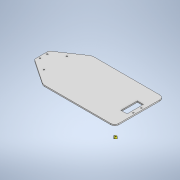
# Autodesk Inventor part: base
Saved by Autodesk Inventor 2020 (Build 240168000, 168)
## iProperties
Created: 2019-08-02
Part Number: base
Material: Generic
Document SubType Name: Modeling
Designer: n10208577
Density: 1 g/cm^3
Appearance: Default
Author: n10208577
Autodesk Inventor part; units mm, degrees
ref_plane "YZ Plane" through (0, 0, 0) normal (1, 0, 0) x (0, 1, 0)
ref_plane "XZ Plane" through (0, 0, 0) normal (0, 1, 0) x (-1, 0, 0)
ref_plane "XY Plane" through (0, 0, 0) normal (0, 0, 1) x (1, 0, 0)
sketch "Sketch1" plane through (0, 0, 0) normal (0, 1, 0) x (-1, 0, 0)
  line L0 (0, 0) -> (0, -28)
  line L1 (0, 0) -> (0, 28)
  circle A0 centre (0, 28) radius 1.6
  circle A1 centre (0, -28) radius 1.6
  line L2 (0, 0) -> (28.5, 0)
  line L3 (28.5, 0) -> (28.5, 8.75)
  line L4 (28.5, 0) -> (28.5, -8.75)
  circle A2 centre (28.5, 8.75) radius 1.6
  circle A3 centre (28.5, -8.75) radius 1.6
  line L5 (-200, 0) -> (-200, -10)
  line L6 (-200, 0) -> (-200, 10)
  circle A4 centre (-200, -10) radius 1.6
  circle A5 centre (-200, 10) radius 1.6
  line L7 (-200, 0) -> (-195, 0)
  line L8 (-195, 0) -> (-195, 20)
  line L9 (-195, 20) -> (-180, 20)
  line L10 (-180, 20) -> (-180, -20)
  line L11 (-180, -20) -> (-195, -20)
  line L12 (-195, -20) -> (-195, 0)
  line L13 (0, 0) -> (-180, 0)
  line L14 (-195, 0) -> (-200, 0)
  line L15 (-200, 0) -> (-205, 0)
  line L16 (-205, 0) -> (-205, 50)
  line L17 (28.5, 8.75) -> (0, 28)
  line L18 (-195, 60) -> (-34.1018, 60)
  line L19 (31.2986, 18.9271) -> (-25.706, 57.4302)
  line L20 (28.5, 8.75) -> (33.5, 8.75)
  line L21 (33.5, 14.7837) -> (33.5, -14.7837)
  line L22 (33.5, -8.75) -> (28.5, -8.75)
  line L23 (-205, 0) -> (-205, -50)
  line L24 (-195, -60) -> (-34.1018, -60)
  line L25 (31.2986, -18.9271) -> (-25.706, -57.4302)
  arc A6 (-25.706, 57.4302) -> (-34.1018, 60) centre (-34.1018, 45) ccw
  arc A7 (-34.1018, -60) -> (-25.706, -57.4302) centre (-34.1018, -45) ccw
  arc A8 (33.5, 14.7837) -> (31.2986, 18.9271) centre (28.5, 14.7837) ccw
  arc A9 (31.2986, -18.9271) -> (33.5, -14.7837) centre (28.5, -14.7837) ccw
  arc A10 (-205, -50) -> (-195, -60) centre (-195, -50) ccw
  arc A11 (-195, 60) -> (-205, 50) centre (-195, 50) ccw
  point P0 (-205, 60)
  point P1 (-29.5106, 60)
  point P2 (36.2986, 15.5499)
  point P3 (-205, -60)
  point P4 (-29.5106, -60)
  point P5 (36.2986, -15.5499)
  point P6 (-206.7664, -60)
  dimension "d0" = 28
  dimension "d1" = 28
  dimension "d2" = 3.2
  dimension "d3" = 3.2
  dimension "d4" = 28.5
  dimension "d5" = 8.75
  dimension "d6" = 8.75
  dimension "d7" = 3.2
  dimension "d8" = 3.2
  dimension "d9" = 200
  dimension "d10" = 10
  dimension "d11" = 10
  dimension "d12" = 3.2
  dimension "d13" = 3.2
  dimension "d14" = 5
  dimension "d15" = 20
  dimension "d16" = 15
  dimension "d17" = 40
  dimension "d18" = 15
  dimension "d19" = 5
  dimension "d21" = 60
  dimension "d23" = 60
  dimension "d24" = 10
  dimension "d25" = 5
  dimension "d28" = 15
  dimension "d29" = 5
  dimension "d30" = 10
  dimension "d31" = 10
  constraints: 52 end point, 16 point on line, 12 centre point, 12 point on circle, 12 tangent, 7 vertical, 6 coincident, 6 horizontal, 6 perpendicular, 3 symmetric about line, 2 equal radius, 1 midpoint, 1 parallel
  measures "d0" distance of L0.start L0.end
  measures "d1" distance of L0.start L1.end
  measures "d2" diameter of A0
  measures "d3" diameter of A1
  measures "d4" distance of L0.start L2.end
  measures "d5" distance of L2.end L3.end
  measures "d6" distance of L2.end L4.end
  measures "d7" diameter of A2
  measures "d8" diameter of A3
  measures "d9" distance of L0.start L5.start
  measures "d10" distance of L5.start L5.end
  measures "d11" distance of L5.start L6.end
  measures "d12" diameter of A4
  measures "d13" diameter of A5
  measures "d14" distance of L5.start L7.end
  measures "d15" distance of L7.end L8.end
  measures "d16" distance of L8.end L9.end
  measures "d17" distance of L9.end L10.end
  measures "d18" distance of L10.end L11.end
  measures "d19" distance of L5.start L15.end
  measures "d21" distance of L15.end point (-205, 60)
  measures "d23" distance between parallel lines of L18 L13
  measures "d24" distance between parallel lines of L17 L19
  measures "d25" distance of L17.start L20.end
  measures "d28" radius of A6
  measures "d29" radius of A8
  measures "d30" radius of A10
  measures "d31" radius of A11
extrude "Extrusion1" add sketch "Sketch1" along normal blind 3 contours L13 L10 L9 L8 L7 L15 L16 A11 L18 A6 L19 A8 L21 L20 A2 L17 A0 L1 | L1 A0 L17 A2 L3 L2 | L2 L4 A3 L22 L21 A9 L25 A7 L24 A10 L23 L15 L7 L12 L11 L10 L13 | L3 A2 L20 L21 L22 A3 L4
body "Solid1"
